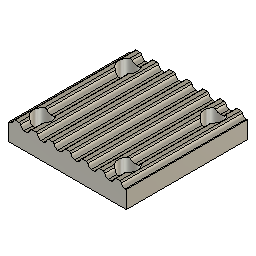
Carriage Rail Belt Clamp (Autodesk Fusion 360 archive; units mm, degrees)
design "TBCR Rail Belt Clamp" references "15mm HTD 5mm Timing Belt Loop"
Autodesk Fusion 360 part; units mm, degrees
(part 1 of 2)
sketch "Sketch1" plane through (0, 0, 0) normal (0, 0, 1) x (1, 0, 0)
  line L0 (17.5, 18) -> (-17.5, 18)
  line L1 (-17.5, 18) -> (-17.5, -18)
  line L2 (-17.5, -18) -> (17.5, -18)
  line L3 (17.5, -18) -> (17.5, 18)
  line L4 (17.5, 18) -> (-17.5, -18) construction
  line L5 (-17.5, 18) -> (17.5, -18) construction
  line L6 (0, 0) -> (0, 18) construction
  line L7 (0, 0) -> (17.5, 0) construction
  line L8 (12.5, 13) -> (-12.5, 13) construction
  line L9 (-12.5, 13) -> (-12.5, -13) construction
  line L10 (-12.5, -13) -> (12.5, -13) construction
  line L11 (12.5, -13) -> (12.5, 13) construction
  line L12 (12.5, 13) -> (-12.5, -13) construction
  line L13 (-12.5, 13) -> (12.5, -13) construction
  circle A0 centre (-12.5, 13) radius 2.25
  circle A1 centre (12.5, 13) radius 2.25
  circle A2 centre (12.5, -13) radius 2.25
  circle A3 centre (-12.5, -13) radius 2.25
  dimension "d10" = 35
  dimension "d11" = 36
  dimension "d13" = 25
  dimension "d14" = 26
  dimension "d15" = 4.5
  constraint horizontal L0
  constraint perpendicular L0 L1
  constraint parallel L0 L2
  constraint parallel L1 L3
  constraint coincident L4 L6.start
  constraint coincident L5 L6.start
  constraint coincident L6.start L7.start
  constraint midpoint L0 L6.end
  constraint midpoint L3 L7.end
  constraint horizontal L8
  constraint perpendicular L8 L9
  constraint parallel L8 L10
  constraint parallel L9 L11
  constraint coincident L12 L6.start
  constraint coincident L13 L6.start
  constraint coincident L8.end L9.start
  constraint coincident L8.start L11.end
  constraint coincident L10.end L11.start
  constraint coincident L9.end L10.start
  constraint equal A0 A3
  constraint equal A0 A2
  constraint equal A1 A2
  measures "d10" distance of L1.end L2.end
  measures "d11" distance of L0.end L1.end
  measures "d13" distance of L9.end L10.end
  measures "d14" distance of L8.end L9.end
  measures "d15" diameter of A0
extrude "Extrude1" add sketch "Sketch1" along normal blind 6.5
sketch "Sketch2" plane through (0, -18, 0) normal (0, -1, 0) x (1, 0, 0)
  line L0 (-17.5, 0) -> (17.5, 0)
  line L1 (17.5, 0) -> (17.5, 6.5)
  line L2 (17.5, 6.5) -> (-17.5, 6.5)
  line L3 (-17.5, 6.5) -> (-17.5, 0)
  arc A0 (-52.5, 8.4003) -> (-52.5, -87.0926) centre (-52.5, -39.3462) ccw
  line L4 (-52.5, -87.0926) -> (47.5, -87.0926)
  arc A1 (47.5, -87.0926) -> (47.5, 8.4003) centre (47.5, -39.3462) ccw
  line L5 (47.5, 8.4003) -> (-52.5, 8.4003)
  arc A2 (49.2562, -85.159) -> (50.5422, -85.0916) centre (47.5, -39.3462) ccw
  arc A3 (48.9524, -84.8176) -> (49.2562, -85.159) centre (49.4365, -84.6926) ccw
  arc A4 (48.9524, -84.8176) -> (47.9167, -83.7517) centre (47.5, -85.1926) ccw
  arc A5 (47.0833, -83.7517) -> (47.9167, -83.7517) centre (47.5, -83.03) ccw
  arc A6 (47.0833, -83.7517) -> (46.0476, -84.8176) centre (47.5, -85.1926) ccw
  arc A7 (45.5635, -85.1926) -> (46.0476, -84.8176) centre (45.5635, -84.6926) ccw
  line L6 (45.5635, -85.1926) -> (44.4365, -85.1926)
  arc A8 (43.9524, -84.8176) -> (44.4365, -85.1926) centre (44.4365, -84.6926) ccw
  arc A9 (43.9524, -84.8176) -> (42.9167, -83.7517) centre (42.5, -85.1926) ccw
  arc A10 (42.0833, -83.7517) -> (42.9167, -83.7517) centre (42.5, -83.03) ccw
  arc A11 (42.0833, -83.7517) -> (41.0476, -84.8176) centre (42.5, -85.1926) ccw
  arc A12 (40.5635, -85.1926) -> (41.0476, -84.8176) centre (40.5635, -84.6926) ccw
  line L7 (40.5635, -85.1926) -> (39.4365, -85.1926)
  arc A13 (38.9524, -84.8176) -> (39.4365, -85.1926) centre (39.4365, -84.6926) ccw
  arc A14 (38.9524, -84.8176) -> (37.9167, -83.7517) centre (37.5, -85.1926) ccw
  arc A15 (37.0833, -83.7517) -> (37.9167, -83.7517) centre (37.5, -83.03) ccw
  arc A16 (37.0833, -83.7517) -> (36.0476, -84.8176) centre (37.5, -85.1926) ccw
  arc A17 (35.5635, -85.1926) -> (36.0476, -84.8176) centre (35.5635, -84.6926) ccw
  line L8 (35.5635, -85.1926) -> (34.4365, -85.1926)
  arc A18 (33.9524, -84.8176) -> (34.4365, -85.1926) centre (34.4365, -84.6926) ccw
  arc A19 (33.9524, -84.8176) -> (32.9167, -83.7517) centre (32.5, -85.1926) ccw
  arc A20 (32.0833, -83.7517) -> (32.9167, -83.7517) centre (32.5, -83.03) ccw
  arc A21 (32.0833, -83.7517) -> (31.0476, -84.8176) centre (32.5, -85.1926) ccw
  arc A22 (30.5635, -85.1926) -> (31.0476, -84.8176) centre (30.5635, -84.6926) ccw
  line L9 (30.5635, -85.1926) -> (29.4365, -85.1926)
  arc A23 (28.9524, -84.8176) -> (29.4365, -85.1926) centre (29.4365, -84.6926) ccw
  arc A24 (28.9524, -84.8176) -> (27.9167, -83.7517) centre (27.5, -85.1926) ccw
  arc A25 (27.0833, -83.7517) -> (27.9167, -83.7517) centre (27.5, -83.03) ccw
  arc A26 (27.0833, -83.7517) -> (26.0476, -84.8176) centre (27.5, -85.1926) ccw
  arc A27 (25.5635, -85.1926) -> (26.0476, -84.8176) centre (25.5635, -84.6926) ccw
  line L10 (25.5635, -85.1926) -> (24.4365, -85.1926)
  arc A28 (23.9524, -84.8176) -> (24.4365, -85.1926) centre (24.4365, -84.6926) ccw
  arc A29 (23.9524, -84.8176) -> (22.9167, -83.7517) centre (22.5, -85.1926) ccw
  arc A30 (22.0833, -83.7517) -> (22.9167, -83.7517) centre (22.5, -83.03) ccw
  arc A31 (22.0833, -83.7517) -> (21.0476, -84.8176) centre (22.5, -85.1926) ccw
  arc A32 (20.5635, -85.1926) -> (21.0476, -84.8176) centre (20.5635, -84.6926) ccw
  line L11 (20.5635, -85.1926) -> (19.4365, -85.1926)
  arc A33 (18.9524, -84.8176) -> (19.4365, -85.1926) centre (19.4365, -84.6926) ccw
  arc A34 (18.9524, -84.8176) -> (17.9167, -83.7517) centre (17.5, -85.1926) ccw
  arc A35 (17.0833, -83.7517) -> (17.9167, -83.7517) centre (17.5, -83.03) ccw
  arc A36 (17.0833, -83.7517) -> (16.0476, -84.8176) centre (17.5, -85.1926) ccw
  arc A37 (15.5635, -85.1926) -> (16.0476, -84.8176) centre (15.5635, -84.6926) ccw
  line L12 (15.5635, -85.1926) -> (14.4365, -85.1926)
  arc A38 (13.9524, -84.8176) -> (14.4365, -85.1926) centre (14.4365, -84.6926) ccw
  arc A39 (13.9524, -84.8176) -> (12.9167, -83.7517) centre (12.5, -85.1926) ccw
  arc A40 (12.0833, -83.7517) -> (12.9167, -83.7517) centre (12.5, -83.03) ccw
  arc A41 (12.0833, -83.7517) -> (11.0476, -84.8176) centre (12.5, -85.1926) ccw
  arc A42 (10.5635, -85.1926) -> (11.0476, -84.8176) centre (10.5635, -84.6926) ccw
  line L13 (10.5635, -85.1926) -> (9.4365, -85.1926)
  arc A43 (8.9524, -84.8176) -> (9.4365, -85.1926) centre (9.4365, -84.6926) ccw
  arc A44 (8.9524, -84.8176) -> (7.9167, -83.7517) centre (7.5, -85.1926) ccw
  arc A45 (7.0833, -83.7517) -> (7.9167, -83.7517) centre (7.5, -83.03) ccw
  arc A46 (7.0833, -83.7517) -> (6.0476, -84.8176) centre (7.5, -85.1926) ccw
  arc A47 (5.5635, -85.1926) -> (6.0476, -84.8176) centre (5.5635, -84.6926) ccw
  line L14 (5.5635, -85.1926) -> (4.4365, -85.1926)
  arc A48 (3.9524, -84.8176) -> (4.4365, -85.1926) centre (4.4365, -84.6926) ccw
  arc A49 (3.9524, -84.8176) -> (2.9167, -83.7517) centre (2.5, -85.1926) ccw
  arc A50 (2.0833, -83.7517) -> (2.9167, -83.7517) centre (2.5, -83.03) ccw
  arc A51 (2.0833, -83.7517) -> (1.0476, -84.8176) centre (2.5, -85.1926) ccw
  arc A52 (0.5635, -85.1926) -> (1.0476, -84.8176) centre (0.5635, -84.6926) ccw
  line L15 (0.5635, -85.1926) -> (-0.5635, -85.1926)
  arc A53 (-1.0476, -84.8176) -> (-0.5635, -85.1926) centre (-0.5635, -84.6926) ccw
  arc A54 (-1.0476, -84.8176) -> (-2.0833, -83.7517) centre (-2.5, -85.1926) ccw
  arc A55 (-2.9167, -83.7517) -> (-2.0833, -83.7517) centre (-2.5, -83.03) ccw
  arc A56 (-2.9167, -83.7517) -> (-3.9524, -84.8176) centre (-2.5, -85.1926) ccw
  arc A57 (-4.4365, -85.1926) -> (-3.9524, -84.8176) centre (-4.4365, -84.6926) ccw
  line L16 (-4.4365, -85.1926) -> (-5.5635, -85.1926)
  arc A58 (-6.0476, -84.8176) -> (-5.5635, -85.1926) centre (-5.5635, -84.6926) ccw
  arc A59 (-6.0476, -84.8176) -> (-7.0833, -83.7517) centre (-7.5, -85.1926) ccw
  arc A60 (-7.9167, -83.7517) -> (-7.0833, -83.7517) centre (-7.5, -83.03) ccw
  arc A61 (-7.9167, -83.7517) -> (-8.9524, -84.8176) centre (-7.5, -85.1926) ccw
  arc A62 (-9.4365, -85.1926) -> (-8.9524, -84.8176) centre (-9.4365, -84.6926) ccw
  line L17 (-9.4365, -85.1926) -> (-10.5635, -85.1926)
  arc A63 (-11.0476, -84.8176) -> (-10.5635, -85.1926) centre (-10.5635, -84.6926) ccw
  arc A64 (-11.0476, -84.8176) -> (-12.0833, -83.7517) centre (-12.5, -85.1926) ccw
  arc A65 (-12.9167, -83.7517) -> (-12.0833, -83.7517) centre (-12.5, -83.03) ccw
  arc A66 (-12.9167, -83.7517) -> (-13.9524, -84.8176) centre (-12.5, -85.1926) ccw
  arc A67 (-14.4365, -85.1926) -> (-13.9524, -84.8176) centre (-14.4365, -84.6926) ccw
  line L18 (-14.4365, -85.1926) -> (-15.5635, -85.1926)
  arc A68 (-16.0476, -84.8176) -> (-15.5635, -85.1926) centre (-15.5635, -84.6926) ccw
  arc A69 (-16.0476, -84.8176) -> (-17.0833, -83.7517) centre (-17.5, -85.1926) ccw
  arc A70 (-17.9167, -83.7517) -> (-17.0833, -83.7517) centre (-17.5, -83.03) ccw
  arc A71 (-17.9167, -83.7517) -> (-18.9524, -84.8176) centre (-17.5, -85.1926) ccw
  arc A72 (-19.4365, -85.1926) -> (-18.9524, -84.8176) centre (-19.4365, -84.6926) ccw
  line L19 (-19.4365, -85.1926) -> (-20.5635, -85.1926)
  arc A73 (-21.0476, -84.8176) -> (-20.5635, -85.1926) centre (-20.5635, -84.6926) ccw
  arc A74 (-21.0476, -84.8176) -> (-22.0833, -83.7517) centre (-22.5, -85.1926) ccw
  arc A75 (-22.9167, -83.7517) -> (-22.0833, -83.7517) centre (-22.5, -83.03) ccw
  arc A76 (-22.9167, -83.7517) -> (-23.9524, -84.8176) centre (-22.5, -85.1926) ccw
  arc A77 (-24.4365, -85.1926) -> (-23.9524, -84.8176) centre (-24.4365, -84.6926) ccw
  line L20 (-24.4365, -85.1926) -> (-25.5635, -85.1926)
  arc A78 (-26.0476, -84.8176) -> (-25.5635, -85.1926) centre (-25.5635, -84.6926) ccw
  arc A79 (-26.0476, -84.8176) -> (-27.0833, -83.7517) centre (-27.5, -85.1926) ccw
  arc A80 (-27.9167, -83.7517) -> (-27.0833, -83.7517) centre (-27.5, -83.03) ccw
  arc A81 (-27.9167, -83.7517) -> (-28.9524, -84.8176) centre (-27.5, -85.1926) ccw
  arc A82 (-29.4365, -85.1926) -> (-28.9524, -84.8176) centre (-29.4365, -84.6926) ccw
  line L21 (-29.4365, -85.1926) -> (-30.5635, -85.1926)
  arc A83 (-31.0476, -84.8176) -> (-30.5635, -85.1926) centre (-30.5635, -84.6926) ccw
  arc A84 (-31.0476, -84.8176) -> (-32.0833, -83.7517) centre (-32.5, -85.1926) ccw
  arc A85 (-32.9167, -83.7517) -> (-32.0833, -83.7517) centre (-32.5, -83.03) ccw
  arc A86 (-32.9167, -83.7517) -> (-33.9524, -84.8176) centre (-32.5, -85.1926) ccw
  arc A87 (-34.4365, -85.1926) -> (-33.9524, -84.8176) centre (-34.4365, -84.6926) ccw
  line L22 (-34.4365, -85.1926) -> (-35.5635, -85.1926)
  arc A88 (-36.0476, -84.8176) -> (-35.5635, -85.1926) centre (-35.5635, -84.6926) ccw
  arc A89 (-36.0476, -84.8176) -> (-37.0833, -83.7517) centre (-37.5, -85.1926) ccw
  arc A90 (-37.9167, -83.7517) -> (-37.0833, -83.7517) centre (-37.5, -83.03) ccw
  arc A91 (-37.9167, -83.7517) -> (-38.9524, -84.8176) centre (-37.5, -85.1926) ccw
  arc A92 (-39.4365, -85.1926) -> (-38.9524, -84.8176) centre (-39.4365, -84.6926) ccw
  line L23 (-39.4365, -85.1926) -> (-40.5635, -85.1926)
  arc A93 (-41.0476, -84.8176) -> (-40.5635, -85.1926) centre (-40.5635, -84.6926) ccw
  arc A94 (-41.0476, -84.8176) -> (-42.0833, -83.7517) centre (-42.5, -85.1926) ccw
  arc A95 (-42.9167, -83.7517) -> (-42.0833, -83.7517) centre (-42.5, -83.03) ccw
  arc A96 (-42.9167, -83.7517) -> (-43.9524, -84.8176) centre (-42.5, -85.1926) ccw
  arc A97 (-44.4365, -85.1926) -> (-43.9524, -84.8176) centre (-44.4365, -84.6926) ccw
  line L24 (-44.4365, -85.1926) -> (-45.5635, -85.1926)
  arc A98 (-46.0476, -84.8176) -> (-45.5635, -85.1926) centre (-45.5635, -84.6926) ccw
  arc A99 (-46.0476, -84.8176) -> (-47.0833, -83.7517) centre (-47.5, -85.1926) ccw
  arc A100 (-47.9167, -83.7517) -> (-47.0833, -83.7517) centre (-47.5, -83.03) ccw
  arc A101 (-47.9167, -83.7517) -> (-48.9524, -84.8176) centre (-47.5, -85.1926) ccw
  arc A102 (-49.4365, -85.1926) -> (-48.9524, -84.8176) centre (-49.4365, -84.6926) ccw
  line L25 (-49.4365, -85.1926) -> (-50.5635, -85.1926)
  arc A103 (-51.0476, -84.8176) -> (-50.5635, -85.1926) centre (-50.5635, -84.6926) ccw
  arc A104 (-51.0476, -84.8176) -> (-52.0833, -83.7517) centre (-52.5, -85.1926) ccw
  arc A105 (-52.9167, -83.7517) -> (-52.0833, -83.7517) centre (-52.5, -83.03) ccw
  arc A106 (-52.9167, -83.7517) -> (-53.9524, -84.8176) centre (-52.5, -85.1926) ccw
  arc A107 (-54.2562, -85.159) -> (-53.9524, -84.8176) centre (-54.4365, -84.6926) ccw
  arc A108 (-55.5422, -85.0916) -> (-54.2562, -85.159) centre (-52.5, -39.3462) ccw
  arc A109 (-55.8087, -84.7204) -> (-55.5422, -85.0916) centre (-55.3141, -84.6466) ccw
  arc A110 (-55.8087, -84.7204) -> (-56.7273, -83.552) centre (-57.2923, -84.9415) ccw
  arc A111 (-57.556, -83.4649) -> (-56.7273, -83.552) centre (-57.0662, -82.7907) ccw
  arc A112 (-57.556, -83.4649) -> (-58.6975, -84.4167) centre (-57.2923, -84.9415) ccw
  arc A113 (-59.0353, -84.7245) -> (-58.6975, -84.4167) centre (-59.1659, -84.2418) ccw
  arc A114 (-60.3072, -84.523) -> (-59.0353, -84.7245) centre (-52.5, -39.3462) ccw
  arc A115 (-60.5334, -84.1259) -> (-60.3072, -84.523) centre (-60.0339, -84.1043) ccw
  arc A116 (-60.5334, -84.1259) -> (-61.3249, -82.8679) centre (-62.032, -84.1908) ccw
  arc A117 (-62.14, -82.6947) -> (-61.3249, -82.8679) centre (-61.5824, -82.0754) ccw
  arc A118 (-62.14, -82.6947) -> (-63.3747, -83.522) centre (-62.032, -84.1908) ccw
  arc A119 (-63.7428, -83.7927) -> (-63.3747, -83.522) centre (-63.8222, -83.2991) ccw
  arc A120 (-64.9867, -83.4594) -> (-63.7428, -83.7927) centre (-52.5, -39.3462) ccw
  arc A121 (-65.1702, -83.0409) -> (-64.9867, -83.4594) centre (-64.6711, -83.0716) ccw
  arc A122 (-65.1702, -83.0409) -> (-65.8258, -81.7071) centre (-66.6673, -82.9488) ccw
  arc A123 (-66.6183, -81.4496) -> (-65.8258, -81.7071) centre (-65.999, -80.8919) ccw
  arc A124 (-66.6183, -81.4496) -> (-67.9327, -82.1433) centre (-66.6673, -82.9488) ccw
  arc A125 (-68.3272, -82.3741) -> (-67.9327, -82.1433) centre (-68.3545, -81.8748) ccw
  arc A126 (-69.5294, -81.9126) -> (-68.3272, -82.3741) centre (-52.5, -39.3462) ccw
  arc A127 (-69.6681, -81.4772) -> (-69.5294, -81.9126) centre (-69.175, -81.5599) ccw
  arc A128 (-69.6681, -81.4772) -> (-70.1807, -80.0821) centre (-71.1474, -81.229) ccw
  arc A129 (-70.942, -79.7431) -> (-70.1807, -80.0821) centre (-70.2678, -79.2533) ccw
  arc A130 (-70.942, -79.7431) -> (-72.3217, -80.2957) centre (-71.1474, -81.229) ccw
  arc A131 (-72.7381, -80.484) -> (-72.3217, -80.2957) centre (-72.7131, -79.9846) ccw
  arc A132 (-73.8855, -79.8993) -> (-72.7381, -80.484) centre (-52.5, -39.3462) ccw
  arc A133 (-73.978, -79.4518) -> (-73.8855, -79.8993) centre (-73.4962, -79.5856) ccw
  arc A134 (-73.978, -79.4518) -> (-74.3419, -78.0108) centre (-75.4232, -79.0504) ccw
  arc A135 (-75.0636, -77.5941) -> (-74.3419, -78.0108) centre (-74.3419, -77.1775) ccw
  arc A136 (-75.0636, -77.5941) -> (-76.4935, -77.9994) centre (-75.4232, -79.0504) ccw
  arc A137 (-76.9273, -78.1432) -> (-76.4935, -77.9994) centre (-76.8503, -77.6491) ccw
  arc A138 (-78.0073, -77.4418) -> (-76.9273, -78.1432) centre (-52.5, -39.3462) ccw
  arc A139 (-78.0525, -76.987) -> (-78.0073, -77.4418) centre (-77.5873, -77.1705) ccw
  arc A140 (-78.0525, -76.987) -> (-78.2638, -75.5159) centre (-79.4479, -76.4367) ccw
  arc A141 (-78.938, -75.0261) -> (-78.2638, -75.5159) centre (-78.1767, -74.6871) ccw
  arc A142 (-78.938, -75.0261) -> (-80.4025, -75.2797) centre (-79.4479, -76.4367) ccw
  arc A143 (-80.8489, -75.3773) -> (-80.4025, -75.2797) centre (-80.7206, -74.894) ccw
  arc A144 (-81.8497, -74.5668) -> (-80.8489, -75.3773) centre (-52.5, -39.3462) ccw
  arc A145 (-81.847, -74.1099) -> (-81.8497, -74.5668) centre (-81.4036, -74.3409) ccw
  arc A146 (-81.847, -74.1099) -> (-81.9034, -72.6247) centre (-83.1773, -73.4167) ccw
  arc A147 (-82.5227, -72.0671) -> (-81.9034, -72.6247) centre (-81.7302, -71.8096) ccw
  arc A148 (-82.5227, -72.0671) -> (-84.0057, -72.1662) centre (-83.1773, -73.4167) ccw
  arc A149 (-84.4599, -72.2166) -> (-84.0057, -72.1662) centre (-84.2818, -71.7494) ccw
  arc A150 (-85.3705, -71.306) -> (-84.4599, -72.2166) centre (-52.5, -39.3462) ccw
  arc A151 (-85.3201, -70.8518) -> (-85.3705, -71.306) centre (-84.9032, -71.128) ccw
  arc A152 (-85.3201, -70.8518) -> (-85.2209, -69.3689) centre (-86.5706, -70.0234) ccw
  arc A153 (-85.7785, -68.7496) -> (-85.2209, -69.3689) centre (-84.9634, -68.5763) ccw
  arc A154 (-85.7785, -68.7496) -> (-87.2637, -68.6932) centre (-86.5706, -70.0234) ccw
  arc A155 (-87.7207, -68.6958) -> (-87.2637, -68.6932) centre (-87.4948, -68.2498) ccw
  arc A156 (-88.5311, -67.695) -> (-87.7207, -68.6958) centre (-52.5, -39.3462) ccw
  arc A157 (-88.4335, -67.2486) -> (-88.5311, -67.695) centre (-88.0478, -67.5668) ccw
  arc A158 (-88.4335, -67.2486) -> (-88.1799, -65.7842) centre (-89.5906, -66.294) ccw
  arc A159 (-88.6697, -65.11) -> (-88.1799, -65.7842) centre (-87.841, -65.0229) ccw
  arc A160 (-88.6697, -65.11) -> (-90.1409, -64.8986) centre (-89.5906, -66.294) ccw
  arc A161 (-90.5956, -64.8535) -> (-90.1409, -64.8986) centre (-90.3243, -64.4335) ccw
  arc A162 (-91.297, -63.7735) -> (-90.5956, -64.8535) centre (-52.5, -39.3462) ccw
  arc A163 (-91.1533, -63.3397) -> (-91.297, -63.7735) centre (-90.803, -63.6965) ccw
  arc A164 (-91.1533, -63.3397) -> (-90.748, -61.9098) centre (-92.2042, -62.2694) ccw
  arc A165 (-91.1646, -61.1881) -> (-90.748, -61.9098) centre (-90.3313, -61.1881) ccw
  arc A166 (-91.1646, -61.1881) -> (-92.6056, -60.8241) centre (-92.2042, -62.2694) ccw
  arc A167 (-93.0532, -60.7317) -> (-92.6056, -60.8241) centre (-92.7395, -60.3424) ccw
  arc A168 (-93.6378, -59.5843) -> (-93.0532, -60.7317) centre (-52.5, -39.3462) ccw
  arc A169 (-93.4495, -59.1679) -> (-93.6378, -59.5843) centre (-93.1384, -59.5593) ccw
  arc A170 (-93.4495, -59.1679) -> (-92.897, -57.7882) centre (-94.3828, -57.9936) ccw
  arc A171 (-93.2359, -57.0269) -> (-92.897, -57.7882) centre (-92.4072, -57.114) ccw
  arc A172 (-93.2359, -57.0269) -> (-94.631, -56.5143) centre (-94.3828, -57.9936) ccw
  arc A173 (-95.0664, -56.3756) -> (-94.631, -56.5143) centre (-94.7137, -56.0212) ccw
  arc A174 (-95.5279, -55.1733) -> (-95.0664, -56.3756) centre (-52.5, -39.3462) ccw
  arc A175 (-95.2971, -54.7789) -> (-95.5279, -55.1733) centre (-95.0287, -55.2007) ccw
  arc A176 (-95.2971, -54.7789) -> (-94.6034, -53.4645) centre (-96.1026, -53.5135) ccw
  arc A177 (-94.8609, -52.6719) -> (-94.6034, -53.4645) centre (-94.0458, -52.8452) ccw
  arc A178 (-94.8609, -52.6719) -> (-96.1948, -52.0163) centre (-96.1026, -53.5135) ccw
  arc A179 (-96.6133, -51.8329) -> (-96.1948, -52.0163) centre (-96.2255, -51.5173) ccw
  arc A180 (-96.9466, -50.589) -> (-96.6133, -51.8329) centre (-52.5, -39.3462) ccw
  arc A181 (-96.6759, -50.2208) -> (-96.9466, -50.589) centre (-96.4529, -50.6684) ccw
  arc A182 (-96.6759, -50.2208) -> (-95.8485, -48.9861) centre (-97.3446, -48.8782) ccw
  arc A183 (-96.0218, -48.171) -> (-95.8485, -48.9861) centre (-95.2292, -48.4285) ccw
  arc A184 (-96.0218, -48.171) -> (-97.2798, -47.3796) centre (-97.3446, -48.8782) ccw
  arc A185 (-97.6768, -47.1534) -> (-97.2798, -47.3796) centre (-97.2582, -46.88) ccw
  arc A186 (-97.8783, -45.8815) -> (-97.6768, -47.1534) centre (-52.5, -39.3462) ccw
  arc A187 (-97.5706, -45.5436) -> (-97.8783, -45.8815) centre (-97.3957, -46.012) ccw
  arc A188 (-97.5706, -45.5436) -> (-96.6187, -44.4022) centre (-98.0953, -44.1384) ccw
  arc A189 (-96.7058, -43.5734) -> (-96.6187, -44.4022) centre (-95.9445, -43.9124) ccw
  arc A190 (-96.7058, -43.5734) -> (-97.8742, -42.6548) centre (-98.0953, -44.1384) ccw
  arc A191 (-98.2454, -42.3884) -> (-97.8742, -42.6548) centre (-97.8005, -42.1603) ccw
  arc A192 (-98.3128, -41.1023) -> (-98.2454, -42.3884) centre (-52.5, -39.3462) ccw
  arc A193 (-97.9715, -40.7985) -> (-98.3128, -41.1023) centre (-97.8465, -41.2827) ccw
  arc A194 (-97.9715, -40.7985) -> (-96.9055, -39.7628) centre (-98.3465, -39.3462) ccw
  arc A195 (-96.9055, -38.9295) -> (-96.9055, -39.7628) centre (-96.1838, -39.3462) ccw
  arc A196 (-96.9055, -38.9295) -> (-97.9715, -37.8938) centre (-98.3465, -39.3462) ccw
  arc A197 (-98.3128, -37.59) -> (-97.9715, -37.8938) centre (-97.8465, -37.4097) ccw
  arc A198 (-98.2454, -36.304) -> (-98.3128, -37.59) centre (-52.5, -39.3462) ccw
  arc A199 (-97.8742, -36.0375) -> (-98.2454, -36.304) centre (-97.8005, -36.532) ccw
  arc A200 (-97.8742, -36.0375) -> (-96.7058, -35.1189) centre (-98.0953, -34.5539) ccw
  arc A201 (-96.6187, -34.2901) -> (-96.7058, -35.1189) centre (-95.9445, -34.78) ccw
  arc A202 (-96.6187, -34.2901) -> (-97.5706, -33.1487) centre (-98.0953, -34.5539) ccw
  arc A203 (-97.8783, -32.8109) -> (-97.5706, -33.1487) centre (-97.3957, -32.6803) ccw
  arc A204 (-97.6768, -31.5389) -> (-97.8783, -32.8109) centre (-52.5, -39.3462) ccw
  arc A205 (-97.2798, -31.3127) -> (-97.6768, -31.5389) centre (-97.2582, -31.8123) ccw
  arc A206 (-97.2798, -31.3127) -> (-96.0218, -30.5213) centre (-97.3446, -29.8141) ccw
  arc A207 (-95.8485, -29.7062) -> (-96.0218, -30.5213) centre (-95.2292, -30.2638) ccw
  arc A208 (-95.8485, -29.7062) -> (-96.6759, -28.4715) centre (-97.3446, -29.8141) ccw
  arc A209 (-96.9466, -28.1033) -> (-96.6759, -28.4715) centre (-96.4529, -28.0239) ccw
  arc A210 (-96.6133, -26.8594) -> (-96.9466, -28.1033) centre (-52.5, -39.3462) ccw
  arc A211 (-96.1948, -26.676) -> (-96.6133, -26.8594) centre (-96.2255, -27.175) ccw
  arc A212 (-96.1948, -26.676) -> (-94.8609, -26.0204) centre (-96.1026, -25.1788) ccw
  arc A213 (-94.6034, -25.2278) -> (-94.8609, -26.0204) centre (-94.0458, -25.8471) ccw
  arc A214 (-94.6034, -25.2278) -> (-95.2971, -23.9134) centre (-96.1026, -25.1788) ccw
  arc A215 (-95.5279, -23.519) -> (-95.2971, -23.9134) centre (-95.0287, -23.4916) ccw
  arc A216 (-95.0664, -22.3167) -> (-95.5279, -23.519) centre (-52.5, -39.3462) ccw
  arc A217 (-94.631, -22.178) -> (-95.0664, -22.3167) centre (-94.7137, -22.6712) ccw
  arc A218 (-94.631, -22.178) -> (-93.2359, -21.6655) centre (-94.3828, -20.6987) ccw
  arc A219 (-92.897, -20.9042) -> (-93.2359, -21.6655) centre (-92.4072, -21.5783) ccw
  arc A220 (-92.897, -20.9042) -> (-93.4495, -19.5244) centre (-94.3828, -20.6987) ccw
  arc A221 (-93.6378, -19.1081) -> (-93.4495, -19.5244) centre (-93.1384, -19.133) ccw
  arc A222 (-93.0532, -17.9606) -> (-93.6378, -19.1081) centre (-52.5, -39.3462) ccw
  arc A223 (-92.6056, -17.8682) -> (-93.0532, -17.9606) centre (-92.7395, -18.35) ccw
  arc A224 (-92.6056, -17.8682) -> (-91.1646, -17.5042) centre (-92.2042, -16.4229) ccw
  arc A225 (-90.748, -16.7826) -> (-91.1646, -17.5042) centre (-90.3313, -17.5042) ccw
  arc A226 (-90.748, -16.7826) -> (-91.1533, -15.3526) centre (-92.2042, -16.4229) ccw
  arc A227 (-91.297, -14.9189) -> (-91.1533, -15.3526) centre (-90.803, -14.9959) ccw
  arc A228 (-90.5956, -13.8388) -> (-91.297, -14.9189) centre (-52.5, -39.3462) ccw
  arc A229 (-90.1409, -13.7937) -> (-90.5956, -13.8388) centre (-90.3243, -14.2588) ccw
  arc A230 (-90.1409, -13.7937) -> (-88.6697, -13.5823) centre (-89.5906, -12.3983) ccw
  arc A231 (-88.1799, -12.9082) -> (-88.6697, -13.5823) centre (-87.841, -13.6695) ccw
  arc A232 (-88.1799, -12.9082) -> (-88.4335, -11.4437) centre (-89.5906, -12.3983) ccw
  arc A233 (-88.5311, -10.9973) -> (-88.4335, -11.4437) centre (-88.0478, -11.1255) ccw
  arc A234 (-87.7207, -9.9965) -> (-88.5311, -10.9973) centre (-52.5, -39.3462) ccw
  arc A235 (-87.2637, -9.9991) -> (-87.7207, -9.9965) centre (-87.4948, -10.4425) ccw
  arc A236 (-87.2637, -9.9991) -> (-85.7785, -9.9427) centre (-86.5706, -8.6689) ccw
  arc A237 (-85.2209, -9.3234) -> (-85.7785, -9.9427) centre (-84.9634, -10.116) ccw
  arc A238 (-85.2209, -9.3234) -> (-85.3201, -7.8405) centre (-86.5706, -8.6689) ccw
  arc A239 (-85.3705, -7.3863) -> (-85.3201, -7.8405) centre (-84.9032, -7.5643) ccw
  arc A240 (-84.4599, -6.4757) -> (-85.3705, -7.3863) centre (-52.5, -39.3462) ccw
  arc A241 (-84.0057, -6.5261) -> (-84.4599, -6.4757) centre (-84.2818, -6.9429) ccw
  arc A242 (-84.0057, -6.5261) -> (-82.5227, -6.6252) centre (-83.1773, -5.2756) ccw
  arc A243 (-81.9034, -6.0676) -> (-82.5227, -6.6252) centre (-81.7302, -6.8828) ccw
  arc A244 (-81.9034, -6.0676) -> (-81.847, -4.5824) centre (-83.1773, -5.2756) ccw
  arc A245 (-81.8497, -4.1255) -> (-81.847, -4.5824) centre (-81.4036, -4.3514) ccw
  arc A246 (-80.8489, -3.315) -> (-81.8497, -4.1255) centre (-52.5, -39.3462) ccw
  arc A247 (-80.4025, -3.4126) -> (-80.8489, -3.315) centre (-80.7206, -3.7983) ccw
  arc A248 (-80.4025, -3.4126) -> (-78.938, -3.6663) centre (-79.4479, -2.2556) ccw
  arc A249 (-78.2638, -3.1764) -> (-78.938, -3.6663) centre (-78.1767, -4.0052) ccw
  arc A250 (-78.2638, -3.1764) -> (-78.0525, -1.7053) centre (-79.4479, -2.2556) ccw
  arc A251 (-78.0073, -1.2505) -> (-78.0525, -1.7053) centre (-77.5873, -1.5218) ccw
  arc A252 (-76.9273, -0.5492) -> (-78.0073, -1.2505) centre (-52.5, -39.3462) ccw
  arc A253 (-76.4935, -0.6929) -> (-76.9273, -0.5492) centre (-76.8503, -1.0432) ccw
  arc A254 (-76.4935, -0.6929) -> (-75.0636, -1.0982) centre (-75.4232, 0.3581) ccw
  arc A255 (-74.3419, -0.6815) -> (-75.0636, -1.0982) centre (-74.3419, -1.5149) ccw
  arc A256 (-74.3419, -0.6815) -> (-73.978, 0.7595) centre (-75.4232, 0.3581) ccw
  arc A257 (-73.8855, 1.207) -> (-73.978, 0.7595) centre (-73.4962, 0.8933) ccw
  arc A258 (-72.7381, 1.7916) -> (-73.8855, 1.207) centre (-52.5, -39.3462) ccw
  arc A259 (-72.3217, 1.6034) -> (-72.7381, 1.7916) centre (-72.7131, 1.2923) ccw
  arc A260 (-72.3217, 1.6034) -> (-70.942, 1.0508) centre (-71.1474, 2.5367) ccw
  arc A261 (-70.1807, 1.3898) -> (-70.942, 1.0508) centre (-70.2678, 0.561) ccw
  arc A262 (-70.1807, 1.3898) -> (-69.6681, 2.7848) centre (-71.1474, 2.5367) ccw
  arc A263 (-69.5294, 3.2202) -> (-69.6681, 2.7848) centre (-69.175, 2.8676) ccw
  arc A264 (-68.3272, 3.6817) -> (-69.5294, 3.2202) centre (-52.5, -39.3462) ccw
  arc A265 (-67.9327, 3.451) -> (-68.3272, 3.6817) centre (-68.3545, 3.1825) ccw
  arc A266 (-67.9327, 3.451) -> (-66.6183, 2.7572) centre (-66.6673, 4.2564) ccw
  arc A267 (-65.8258, 3.0148) -> (-66.6183, 2.7572) centre (-65.999, 2.1996) ccw
  arc A268 (-65.8258, 3.0148) -> (-65.1702, 4.3486) centre (-66.6673, 4.2564) ccw
  arc A269 (-64.9867, 4.7671) -> (-65.1702, 4.3486) centre (-64.6711, 4.3793) ccw
  arc A270 (-63.7428, 5.1004) -> (-64.9867, 4.7671) centre (-52.5, -39.3462) ccw
  arc A271 (-63.3747, 4.8297) -> (-63.7428, 5.1004) centre (-63.8222, 4.6068) ccw
  arc A272 (-63.3747, 4.8297) -> (-62.14, 4.0024) centre (-62.032, 5.4985) ccw
  arc A273 (-61.3249, 4.1756) -> (-62.14, 4.0024) centre (-61.5824, 3.3831) ccw
  arc A274 (-61.3249, 4.1756) -> (-60.5334, 5.4336) centre (-62.032, 5.4985) ccw
  arc A275 (-60.3072, 5.8307) -> (-60.5334, 5.4336) centre (-60.0339, 5.412) ccw
  arc A276 (-59.0353, 6.0321) -> (-60.3072, 5.8307) centre (-52.5, -39.3462) ccw
  arc A277 (-58.6975, 5.7244) -> (-59.0353, 6.0321) centre (-59.1659, 5.5495) ccw
  arc A278 (-58.6975, 5.7244) -> (-57.556, 4.7725) centre (-57.2923, 6.2492) ccw
  arc A279 (-56.7273, 4.8596) -> (-57.556, 4.7725) centre (-57.0662, 4.0984) ccw
  arc A280 (-56.7273, 4.8596) -> (-55.8087, 6.028) centre (-57.2923, 6.2492) ccw
  arc A281 (-55.5422, 6.3993) -> (-55.8087, 6.028) centre (-55.3141, 5.9543) ccw
  arc A282 (-54.2562, 6.4667) -> (-55.5422, 6.3993) centre (-52.5, -39.3462) ccw
  arc A283 (-53.9524, 6.1253) -> (-54.2562, 6.4667) centre (-54.4365, 6.0003) ccw
  arc A284 (-53.9524, 6.1253) -> (-52.9167, 5.0594) centre (-52.5, 6.5003) ccw
  arc A285 (-52.0833, 5.0594) -> (-52.9167, 5.0594) centre (-52.5, 4.3377) ccw
  arc A286 (-52.0833, 5.0594) -> (-51.0476, 6.1253) centre (-52.5, 6.5003) ccw
  arc A287 (-50.5635, 6.5003) -> (-51.0476, 6.1253) centre (-50.5635, 6.0003) ccw
  line L26 (-50.5635, 6.5003) -> (-49.4365, 6.5003)
  arc A288 (-48.9524, 6.1253) -> (-49.4365, 6.5003) centre (-49.4365, 6.0003) ccw
  arc A289 (-48.9524, 6.1253) -> (-47.9167, 5.0594) centre (-47.5, 6.5003) ccw
  arc A290 (-47.0833, 5.0594) -> (-47.9167, 5.0594) centre (-47.5, 4.3377) ccw
  arc A291 (-47.0833, 5.0594) -> (-46.0476, 6.1253) centre (-47.5, 6.5003) ccw
  arc A292 (-45.5635, 6.5003) -> (-46.0476, 6.1253) centre (-45.5635, 6.0003) ccw
  line L27 (-45.5635, 6.5003) -> (-44.4365, 6.5003)
  arc A293 (-43.9524, 6.1253) -> (-44.4365, 6.5003) centre (-44.4365, 6.0003) ccw
  arc A294 (-43.9524, 6.1253) -> (-42.9167, 5.0594) centre (-42.5, 6.5003) ccw
  arc A295 (-42.0833, 5.0594) -> (-42.9167, 5.0594) centre (-42.5, 4.3377) ccw
  arc A296 (-42.0833, 5.0594) -> (-41.0476, 6.1253) centre (-42.5, 6.5003) ccw
  arc A297 (-40.5635, 6.5003) -> (-41.0476, 6.1253) centre (-40.5635, 6.0003) ccw
  line L28 (-40.5635, 6.5003) -> (-39.4365, 6.5003)
  arc A298 (-38.9524, 6.1253) -> (-39.4365, 6.5003) centre (-39.4365, 6.0003) ccw
  arc A299 (-38.9524, 6.1253) -> (-37.9167, 5.0594) centre (-37.5, 6.5003) ccw
  arc A300 (-37.0833, 5.0594) -> (-37.9167, 5.0594) centre (-37.5, 4.3377) ccw
  arc A301 (-37.0833, 5.0594) -> (-36.0476, 6.1253) centre (-37.5, 6.5003) ccw
  arc A302 (-35.5635, 6.5003) -> (-36.0476, 6.1253) centre (-35.5635, 6.0003) ccw
  line L29 (-35.5635, 6.5003) -> (-34.4365, 6.5003)
  arc A303 (-33.9524, 6.1253) -> (-34.4365, 6.5003) centre (-34.4365, 6.0003) ccw
  arc A304 (-33.9524, 6.1253) -> (-32.9167, 5.0594) centre (-32.5, 6.5003) ccw
  arc A305 (-32.0833, 5.0594) -> (-32.9167, 5.0594) centre (-32.5, 4.3377) ccw
  arc A306 (-32.0833, 5.0594) -> (-31.0476, 6.1253) centre (-32.5, 6.5003) ccw
  arc A307 (-30.5635, 6.5003) -> (-31.0476, 6.1253) centre (-30.5635, 6.0003) ccw
  line L30 (-30.5635, 6.5003) -> (-29.4365, 6.5003)
  arc A308 (-28.9524, 6.1253) -> (-29.4365, 6.5003) centre (-29.4365, 6.0003) ccw
  arc A309 (-28.9524, 6.1253) -> (-27.9167, 5.0594) centre (-27.5, 6.5003) ccw
  arc A310 (-27.0833, 5.0594) -> (-27.9167, 5.0594) centre (-27.5, 4.3377) ccw
  arc A311 (-27.0833, 5.0594) -> (-26.0476, 6.1253) centre (-27.5, 6.5003) ccw
  arc A312 (-25.5635, 6.5003) -> (-26.0476, 6.1253) centre (-25.5635, 6.0003) ccw
  line L31 (-25.5635, 6.5003) -> (-24.4365, 6.5003)
  arc A313 (-23.9524, 6.1253) -> (-24.4365, 6.5003) centre (-24.4365, 6.0003) ccw
  arc A314 (-23.9524, 6.1253) -> (-22.9167, 5.0594) centre (-22.5, 6.5003) ccw
  arc A315 (-22.0833, 5.0594) -> (-22.9167, 5.0594) centre (-22.5, 4.3377) ccw
  arc A316 (-22.0833, 5.0594) -> (-21.0476, 6.1253) centre (-22.5, 6.5003) ccw
  arc A317 (-20.5635, 6.5003) -> (-21.0476, 6.1253) centre (-20.5635, 6.0003) ccw
  line L32 (-20.5635, 6.5003) -> (-19.4365, 6.5003)
  arc A318 (-18.9524, 6.1253) -> (-19.4365, 6.5003) centre (-19.4365, 6.0003) ccw
  arc A319 (-18.9524, 6.1253) -> (-17.9167, 5.0594) centre (-17.5, 6.5003) ccw
  arc A320 (-17.0833, 5.0594) -> (-17.9167, 5.0594) centre (-17.5, 4.3377) ccw
  arc A321 (-17.0833, 5.0594) -> (-16.0476, 6.1253) centre (-17.5, 6.5003) ccw
  arc A322 (-15.5635, 6.5003) -> (-16.0476, 6.1253) centre (-15.5635, 6.0003) ccw
  line L33 (-15.5635, 6.5003) -> (-14.4365, 6.5003)
  arc A323 (-13.9524, 6.1253) -> (-14.4365, 6.5003) centre (-14.4365, 6.0003) ccw
  arc A324 (-13.9524, 6.1253) -> (-12.9167, 5.0594) centre (-12.5, 6.5003) ccw
  arc A325 (-12.0833, 5.0594) -> (-12.9167, 5.0594) centre (-12.5, 4.3377) ccw
  arc A326 (-12.0833, 5.0594) -> (-11.0476, 6.1253) centre (-12.5, 6.5003) ccw
  arc A327 (-10.5635, 6.5003) -> (-11.0476, 6.1253) centre (-10.5635, 6.0003) ccw
  line L34 (-10.5635, 6.5003) -> (-9.4365, 6.5003)
  arc A328 (-8.9524, 6.1253) -> (-9.4365, 6.5003) centre (-9.4365, 6.0003) ccw
  arc A329 (-8.9524, 6.1253) -> (-7.9167, 5.0594) centre (-7.5, 6.5003) ccw
  arc A330 (-7.0833, 5.0594) -> (-7.9167, 5.0594) centre (-7.5, 4.3377) ccw
  arc A331 (-7.0833, 5.0594) -> (-6.0476, 6.1253) centre (-7.5, 6.5003) ccw
  arc A332 (-5.5635, 6.5003) -> (-6.0476, 6.1253) centre (-5.5635, 6.0003) ccw
  line L35 (-5.5635, 6.5003) -> (-4.4365, 6.5003)
  arc A333 (-3.9524, 6.1253) -> (-4.4365, 6.5003) centre (-4.4365, 6.0003) ccw
  arc A334 (-3.9524, 6.1253) -> (-2.9167, 5.0594) centre (-2.5, 6.5003) ccw
  arc A335 (-2.0833, 5.0594) -> (-2.9167, 5.0594) centre (-2.5, 4.3377) ccw
  arc A336 (-2.0833, 5.0594) -> (-1.0476, 6.1253) centre (-2.5, 6.5003) ccw
  arc A337 (-0.5635, 6.5003) -> (-1.0476, 6.1253) centre (-0.5635, 6.0003) ccw
  line L36 (-0.5635, 6.5003) -> (0.5635, 6.5003)
  arc A338 (1.0476, 6.1253) -> (0.5635, 6.5003) centre (0.5635, 6.0003) ccw
  arc A339 (1.0476, 6.1253) -> (2.0833, 5.0594) centre (2.5, 6.5003) ccw
  arc A340 (2.9167, 5.0594) -> (2.0833, 5.0594) centre (2.5, 4.3377) ccw
  arc A341 (2.9167, 5.0594) -> (3.9524, 6.1253) centre (2.5, 6.5003) ccw
  arc A342 (4.4365, 6.5003) -> (3.9524, 6.1253) centre (4.4365, 6.0003) ccw
  line L37 (4.4365, 6.5003) -> (5.5635, 6.5003)
  arc A343 (6.0476, 6.1253) -> (5.5635, 6.5003) centre (5.5635, 6.0003) ccw
  arc A344 (6.0476, 6.1253) -> (7.0833, 5.0594) centre (7.5, 6.5003) ccw
  arc A345 (7.9167, 5.0594) -> (7.0833, 5.0594) centre (7.5, 4.3377) ccw
  arc A346 (7.9167, 5.0594) -> (8.9524, 6.1253) centre (7.5, 6.5003) ccw
  arc A347 (9.4365, 6.5003) -> (8.9524, 6.1253) centre (9.4365, 6.0003) ccw
  line L38 (9.4365, 6.5003) -> (10.5635, 6.5003)
  arc A348 (11.0476, 6.1253) -> (10.5635, 6.5003) centre (10.5635, 6.0003) ccw
  arc A349 (11.0476, 6.1253) -> (12.0833, 5.0594) centre (12.5, 6.5003) ccw
  arc A350 (12.9167, 5.0594) -> (12.0833, 5.0594) centre (12.5, 4.3377) ccw
  arc A351 (12.9167, 5.0594) -> (13.9524, 6.1253) centre (12.5, 6.5003) ccw
  arc A352 (14.4365, 6.5003) -> (13.9524, 6.1253) centre (14.4365, 6.0003) ccw
  line L39 (14.4365, 6.5003) -> (15.5635, 6.5003)
  arc A353 (16.0476, 6.1253) -> (15.5635, 6.5003) centre (15.5635, 6.0003) ccw
  arc A354 (16.0476, 6.1253) -> (17.0833, 5.0594) centre (17.5, 6.5003) ccw
  arc A355 (17.9167, 5.0594) -> (17.0833, 5.0594) centre (17.5, 4.3377) ccw
  arc A356 (17.9167, 5.0594) -> (18.9524, 6.1253) centre (17.5, 6.5003) ccw
  arc A357 (19.4365, 6.5003) -> (18.9524, 6.1253) centre (19.4365, 6.0003) ccw
  line L40 (19.4365, 6.5003) -> (20.5635, 6.5003)
  arc A358 (21.0476, 6.1253) -> (20.5635, 6.5003) centre (20.5635, 6.0003) ccw
  arc A359 (21.0476, 6.1253) -> (22.0833, 5.0594) centre (22.5, 6.5003) ccw
  arc A360 (22.9167, 5.0594) -> (22.0833, 5.0594) centre (22.5, 4.3377) ccw
  arc A361 (22.9167, 5.0594) -> (23.9524, 6.1253) centre (22.5, 6.5003) ccw
  arc A362 (24.4365, 6.5003) -> (23.9524, 6.1253) centre (24.4365, 6.0003) ccw
  line L41 (24.4365, 6.5003) -> (25.5635, 6.5003)
  arc A363 (26.0476, 6.1253) -> (25.5635, 6.5003) centre (25.5635, 6.0003) ccw
  arc A364 (26.0476, 6.1253) -> (27.0833, 5.0594) centre (27.5, 6.5003) ccw
  arc A365 (27.9167, 5.0594) -> (27.0833, 5.0594) centre (27.5, 4.3377) ccw
  arc A366 (27.9167, 5.0594) -> (28.9524, 6.1253) centre (27.5, 6.5003) ccw
  arc A367 (29.4365, 6.5003) -> (28.9524, 6.1253) centre (29.4365, 6.0003) ccw
  line L42 (29.4365, 6.5003) -> (30.5635, 6.5003)
  arc A368 (31.0476, 6.1253) -> (30.5635, 6.5003) centre (30.5635, 6.0003) ccw
  arc A369 (31.0476, 6.1253) -> (32.0833, 5.0594) centre (32.5, 6.5003) ccw
  arc A370 (32.9167, 5.0594) -> (32.0833, 5.0594) centre (32.5, 4.3377) ccw
  arc A371 (32.9167, 5.0594) -> (33.9524, 6.1253) centre (32.5, 6.5003) ccw
  arc A372 (34.4365, 6.5003) -> (33.9524, 6.1253) centre (34.4365, 6.0003) ccw
  line L43 (34.4365, 6.5003) -> (35.5635, 6.5003)
  arc A373 (36.0476, 6.1253) -> (35.5635, 6.5003) centre (35.5635, 6.0003) ccw
  arc A374 (36.0476, 6.1253) -> (37.0833, 5.0594) centre (37.5, 6.5003) ccw
  arc A375 (37.9167, 5.0594) -> (37.0833, 5.0594) centre (37.5, 4.3377) ccw
  arc A376 (37.9167, 5.0594) -> (38.9524, 6.1253) centre (37.5, 6.5003) ccw
  arc A377 (39.4365, 6.5003) -> (38.9524, 6.1253) centre (39.4365, 6.0003) ccw
  line L44 (39.4365, 6.5003) -> (40.5635, 6.5003)
  arc A378 (41.0476, 6.1253) -> (40.5635, 6.5003) centre (40.5635, 6.0003) ccw
  arc A379 (41.0476, 6.1253) -> (42.0833, 5.0594) centre (42.5, 6.5003) ccw
  arc A380 (42.9167, 5.0594) -> (42.0833, 5.0594) centre (42.5, 4.3377) ccw
  arc A381 (42.9167, 5.0594) -> (43.9524, 6.1253) centre (42.5, 6.5003) ccw
  arc A382 (44.4365, 6.5003) -> (43.9524, 6.1253) centre (44.4365, 6.0003) ccw
  line L45 (44.4365, 6.5003) -> (45.5635, 6.5003)
  arc A383 (46.0476, 6.1253) -> (45.5635, 6.5003) centre (45.5635, 6.0003) ccw
  arc A384 (46.0476, 6.1253) -> (47.0833, 5.0594) centre (47.5, 6.5003) ccw
  arc A385 (47.9167, 5.0594) -> (47.0833, 5.0594) centre (47.5, 4.3377) ccw
  arc A386 (47.9167, 5.0594) -> (48.9524, 6.1253) centre (47.5, 6.5003) ccw
  arc A387 (49.2562, 6.4667) -> (48.9524, 6.1253) centre (49.4365, 6.0003) ccw
  arc A388 (50.5422, 6.3993) -> (49.2562, 6.4667) centre (47.5, -39.3462) ccw
  arc A389 (50.8087, 6.028) -> (50.5422, 6.3993) centre (50.3141, 5.9543) ccw
  arc A390 (50.8087, 6.028) -> (51.7273, 4.8596) centre (52.2923, 6.2492) ccw
  arc A391 (52.556, 4.7725) -> (51.7273, 4.8596) centre (52.0662, 4.0984) ccw
  arc A392 (52.556, 4.7725) -> (53.6975, 5.7244) centre (52.2923, 6.2492) ccw
  arc A393 (54.0353, 6.0321) -> (53.6975, 5.7244) centre (54.1659, 5.5495) ccw
  arc A394 (55.3072, 5.8307) -> (54.0353, 6.0321) centre (47.5, -39.3462) ccw
  arc A395 (55.5334, 5.4336) -> (55.3072, 5.8307) centre (55.0339, 5.412) ccw
  arc A396 (55.5334, 5.4336) -> (56.3249, 4.1756) centre (57.032, 5.4985) ccw
  arc A397 (57.14, 4.0024) -> (56.3249, 4.1756) centre (56.5824, 3.3831) ccw
  arc A398 (57.14, 4.0024) -> (58.3747, 4.8297) centre (57.032, 5.4985) ccw
  arc A399 (58.7428, 5.1004) -> (58.3747, 4.8297) centre (58.8222, 4.6068) ccw
  arc A400 (59.9867, 4.7671) -> (58.7428, 5.1004) centre (47.5, -39.3462) ccw
  arc A401 (60.1702, 4.3486) -> (59.9867, 4.7671) centre (59.6711, 4.3793) ccw
  arc A402 (60.1702, 4.3486) -> (60.8258, 3.0148) centre (61.6673, 4.2564) ccw
  arc A403 (61.6183, 2.7572) -> (60.8258, 3.0148) centre (60.999, 2.1996) ccw
  arc A404 (61.6183, 2.7572) -> (62.9327, 3.451) centre (61.6673, 4.2564) ccw
  arc A405 (63.3272, 3.6817) -> (62.9327, 3.451) centre (63.3545, 3.1825) ccw
  arc A406 (64.5294, 3.2202) -> (63.3272, 3.6817) centre (47.5, -39.3462) ccw
  arc A407 (64.6681, 2.7848) -> (64.5294, 3.2202) centre (64.175, 2.8676) ccw
  arc A408 (64.6681, 2.7848) -> (65.1807, 1.3898) centre (66.1474, 2.5367) ccw
  arc A409 (65.942, 1.0508) -> (65.1807, 1.3898) centre (65.2678, 0.561) ccw
  arc A410 (65.942, 1.0508) -> (67.3217, 1.6034) centre (66.1474, 2.5367) ccw
  arc A411 (67.7381, 1.7916) -> (67.3217, 1.6034) centre (67.7131, 1.2923) ccw
  arc A412 (68.8855, 1.207) -> (67.7381, 1.7916) centre (47.5, -39.3462) ccw
  arc A413 (68.978, 0.7595) -> (68.8855, 1.207) centre (68.4962, 0.8933) ccw
  arc A414 (68.978, 0.7595) -> (69.3419, -0.6815) centre (70.4232, 0.3581) ccw
  arc A415 (70.0636, -1.0982) -> (69.3419, -0.6815) centre (69.3419, -1.5149) ccw
  arc A416 (70.0636, -1.0982) -> (71.4935, -0.6929) centre (70.4232, 0.3581) ccw
  arc A417 (71.9273, -0.5492) -> (71.4935, -0.6929) centre (71.8503, -1.0432) ccw
  arc A418 (73.0073, -1.2505) -> (71.9273, -0.5492) centre (47.5, -39.3462) ccw
  arc A419 (73.0525, -1.7053) -> (73.0073, -1.2505) centre (72.5873, -1.5218) ccw
  arc A420 (73.0525, -1.7053) -> (73.2638, -3.1764) centre (74.4479, -2.2556) ccw
  arc A421 (73.938, -3.6663) -> (73.2638, -3.1764) centre (73.1767, -4.0052) ccw
  arc A422 (73.938, -3.6663) -> (75.4025, -3.4126) centre (74.4479, -2.2556) ccw
  arc A423 (75.8489, -3.315) -> (75.4025, -3.4126) centre (75.7206, -3.7983) ccw
  arc A424 (76.8497, -4.1255) -> (75.8489, -3.315) centre (47.5, -39.3462) ccw
  arc A425 (76.847, -4.5824) -> (76.8497, -4.1255) centre (76.4036, -4.3514) ccw
  arc A426 (76.847, -4.5824) -> (76.9034, -6.0676) centre (78.1773, -5.2756) ccw
  arc A427 (77.5227, -6.6252) -> (76.9034, -6.0676) centre (76.7302, -6.8828) ccw
  arc A428 (77.5227, -6.6252) -> (79.0057, -6.5261) centre (78.1773, -5.2756) ccw
  arc A429 (79.4599, -6.4757) -> (79.0057, -6.5261) centre (79.2818, -6.9429) ccw
  arc A430 (80.3705, -7.3863) -> (79.4599, -6.4757) centre (47.5, -39.3462) ccw
  arc A431 (80.3201, -7.8405) -> (80.3705, -7.3863) centre (79.9032, -7.5643) ccw
  arc A432 (80.3201, -7.8405) -> (80.2209, -9.3234) centre (81.5706, -8.6689) ccw
  arc A433 (80.7785, -9.9427) -> (80.2209, -9.3234) centre (79.9634, -10.116) ccw
  arc A434 (80.7785, -9.9427) -> (82.2637, -9.9991) centre (81.5706, -8.6689) ccw
  arc A435 (82.7207, -9.9965) -> (82.2637, -9.9991) centre (82.4948, -10.4425) ccw
  arc A436 (83.5311, -10.9973) -> (82.7207, -9.9965) centre (47.5, -39.3462) ccw
  arc A437 (83.4335, -11.4437) -> (83.5311, -10.9973) centre (83.0478, -11.1255) ccw
  arc A438 (83.4335, -11.4437) -> (83.1799, -12.9082) centre (84.5906, -12.3983) ccw
  arc A439 (83.6697, -13.5823) -> (83.1799, -12.9082) centre (82.841, -13.6695) ccw
  arc A440 (83.6697, -13.5823) -> (85.1409, -13.7937) centre (84.5906, -12.3983) ccw
  arc A441 (85.5956, -13.8388) -> (85.1409, -13.7937) centre (85.3243, -14.2588) ccw
  arc A442 (86.297, -14.9189) -> (85.5956, -13.8388) centre (47.5, -39.3462) ccw
  arc A443 (86.1533, -15.3526) -> (86.297, -14.9189) centre (85.803, -14.9959) ccw
  arc A444 (86.1533, -15.3526) -> (85.748, -16.7826) centre (87.2042, -16.4229) ccw
  arc A445 (86.1646, -17.5042) -> (85.748, -16.7826) centre (85.3313, -17.5042) ccw
  arc A446 (86.1646, -17.5042) -> (87.6056, -17.8682) centre (87.2042, -16.4229) ccw
  arc A447 (88.0532, -17.9606) -> (87.6056, -17.8682) centre (87.7395, -18.35) ccw
  arc A448 (88.6378, -19.1081) -> (88.0532, -17.9606) centre (47.5, -39.3462) ccw
  arc A449 (88.4495, -19.5244) -> (88.6378, -19.1081) centre (88.1384, -19.133) ccw
  arc A450 (88.4495, -19.5244) -> (87.897, -20.9042) centre (89.3828, -20.6987) ccw
  arc A451 (88.2359, -21.6655) -> (87.897, -20.9042) centre (87.4072, -21.5783) ccw
  arc A452 (88.2359, -21.6655) -> (89.631, -22.178) centre (89.3828, -20.6987) ccw
  arc A453 (90.0664, -22.3167) -> (89.631, -22.178) centre (89.7137, -22.6712) ccw
  arc A454 (90.5279, -23.519) -> (90.0664, -22.3167) centre (47.5, -39.3462) ccw
  arc A455 (90.2971, -23.9134) -> (90.5279, -23.519) centre (90.0287, -23.4916) ccw
  arc A456 (90.2971, -23.9134) -> (89.6034, -25.2278) centre (91.1026, -25.1788) ccw
  arc A457 (89.8609, -26.0204) -> (89.6034, -25.2278) centre (89.0458, -25.8471) ccw
  arc A458 (89.8609, -26.0204) -> (91.1948, -26.676) centre (91.1026, -25.1788) ccw
  arc A459 (91.6133, -26.8594) -> (91.1948, -26.676) centre (91.2255, -27.175) ccw
  arc A460 (91.9466, -28.1033) -> (91.6133, -26.8594) centre (47.5, -39.3462) ccw
  arc A461 (91.6759, -28.4715) -> (91.9466, -28.1033) centre (91.4529, -28.0239) ccw
  arc A462 (91.6759, -28.4715) -> (90.8485, -29.7062) centre (92.3446, -29.8141) ccw
  arc A463 (91.0218, -30.5213) -> (90.8485, -29.7062) centre (90.2292, -30.2638) ccw
  arc A464 (91.0218, -30.5213) -> (92.2798, -31.3127) centre (92.3446, -29.8141) ccw
  arc A465 (92.6768, -31.5389) -> (92.2798, -31.3127) centre (92.2582, -31.8123) ccw
  arc A466 (92.8783, -32.8109) -> (92.6768, -31.5389) centre (47.5, -39.3462) ccw
  arc A467 (92.5706, -33.1487) -> (92.8783, -32.8109) centre (92.3957, -32.6803) ccw
  arc A468 (92.5706, -33.1487) -> (91.6187, -34.2901) centre (93.0953, -34.5539) ccw
  arc A469 (91.7058, -35.1189) -> (91.6187, -34.2901) centre (90.9445, -34.78) ccw
  arc A470 (91.7058, -35.1189) -> (92.8742, -36.0375) centre (93.0953, -34.5539) ccw
  arc A471 (93.2454, -36.304) -> (92.8742, -36.0375) centre (92.8005, -36.532) ccw
  arc A472 (93.3128, -37.59) -> (93.2454, -36.304) centre (47.5, -39.3462) ccw
  arc A473 (92.9715, -37.8938) -> (93.3128, -37.59) centre (92.8465, -37.4097) ccw
  arc A474 (92.9715, -37.8938) -> (91.9055, -38.9295) centre (93.3465, -39.3462) ccw
  arc A475 (91.9055, -39.7628) -> (91.9055, -38.9295) centre (91.1838, -39.3462) ccw
  arc A476 (91.9055, -39.7628) -> (92.9715, -40.7985) centre (93.3465, -39.3462) ccw
  arc A477 (93.3128, -41.1023) -> (92.9715, -40.7985) centre (92.8465, -41.2827) ccw
  arc A478 (93.2454, -42.3884) -> (93.3128, -41.1023) centre (47.5, -39.3462) ccw
  arc A479 (92.8742, -42.6548) -> (93.2454, -42.3884) centre (92.8005, -42.1603) ccw
  arc A480 (92.8742, -42.6548) -> (91.7058, -43.5734) centre (93.0953, -44.1384) ccw
  arc A481 (91.6187, -44.4022) -> (91.7058, -43.5734) centre (90.9445, -43.9124) ccw
  arc A482 (91.6187, -44.4022) -> (92.5706, -45.5436) centre (93.0953, -44.1384) ccw
  arc A483 (92.8783, -45.8815) -> (92.5706, -45.5436) centre (92.3957, -46.012) ccw
  arc A484 (92.6768, -47.1534) -> (92.8783, -45.8815) centre (47.5, -39.3462) ccw
  arc A485 (92.2798, -47.3796) -> (92.6768, -47.1534) centre (92.2582, -46.88) ccw
  arc A486 (92.2798, -47.3796) -> (91.0218, -48.171) centre (92.3446, -48.8782) ccw
  arc A487 (90.8485, -48.9861) -> (91.0218, -48.171) centre (90.2292, -48.4285) ccw
  arc A488 (90.8485, -48.9861) -> (91.6759, -50.2208) centre (92.3446, -48.8782) ccw
  arc A489 (91.9466, -50.589) -> (91.6759, -50.2208) centre (91.4529, -50.6684) ccw
  arc A490 (91.6133, -51.8329) -> (91.9466, -50.589) centre (47.5, -39.3462) ccw
  arc A491 (91.1948, -52.0163) -> (91.6133, -51.8329) centre (91.2255, -51.5173) ccw
  arc A492 (91.1948, -52.0163) -> (89.8609, -52.6719) centre (91.1026, -53.5135) ccw
  arc A493 (89.6034, -53.4645) -> (89.8609, -52.6719) centre (89.0458, -52.8452) ccw
  arc A494 (89.6034, -53.4645) -> (90.2971, -54.7789) centre (91.1026, -53.5135) ccw
  arc A495 (90.5279, -55.1733) -> (90.2971, -54.7789) centre (90.0287, -55.2007) ccw
  arc A496 (90.0664, -56.3756) -> (90.5279, -55.1733) centre (47.5, -39.3462) ccw
  arc A497 (89.631, -56.5143) -> (90.0664, -56.3756) centre (89.7137, -56.0212) ccw
  arc A498 (89.631, -56.5143) -> (88.2359, -57.0269) centre (89.3828, -57.9936) ccw
  arc A499 (87.897, -57.7882) -> (88.2359, -57.0269) centre (87.4072, -57.114) ccw
  arc A500 (87.897, -57.7882) -> (88.4495, -59.1679) centre (89.3828, -57.9936) ccw
  arc A501 (88.6378, -59.5843) -> (88.4495, -59.1679) centre (88.1384, -59.5593) ccw
  arc A502 (88.0532, -60.7317) -> (88.6378, -59.5843) centre (47.5, -39.3462) ccw
  arc A503 (87.6056, -60.8241) -> (88.0532, -60.7317) centre (87.7395, -60.3424) ccw
  arc A504 (87.6056, -60.8241) -> (86.1646, -61.1881) centre (87.2042, -62.2694) ccw
  arc A505 (85.748, -61.9098) -> (86.1646, -61.1881) centre (85.3313, -61.1881) ccw
  arc A506 (85.748, -61.9098) -> (86.1533, -63.3397) centre (87.2042, -62.2694) ccw
  arc A507 (86.297, -63.7735) -> (86.1533, -63.3397) centre (85.803, -63.6965) ccw
  arc A508 (85.5956, -64.8535) -> (86.297, -63.7735) centre (47.5, -39.3462) ccw
  arc A509 (85.1409, -64.8986) -> (85.5956, -64.8535) centre (85.3243, -64.4335) ccw
  arc A510 (85.1409, -64.8986) -> (83.6697, -65.11) centre (84.5906, -66.294) ccw
  arc A511 (83.1799, -65.7842) -> (83.6697, -65.11) centre (82.841, -65.0229) ccw
  arc A512 (83.1799, -65.7842) -> (83.4335, -67.2486) centre (84.5906, -66.294) ccw
  arc A513 (83.5311, -67.695) -> (83.4335, -67.2486) centre (83.0478, -67.5668) ccw
  arc A514 (82.7207, -68.6958) -> (83.5311, -67.695) centre (47.5, -39.3462) ccw
  arc A515 (82.2637, -68.6932) -> (82.7207, -68.6958) centre (82.4948, -68.2498) ccw
  arc A516 (82.2637, -68.6932) -> (80.7785, -68.7496) centre (81.5706, -70.0234) ccw
  arc A517 (80.2209, -69.3689) -> (80.7785, -68.7496) centre (79.9634, -68.5763) ccw
  arc A518 (80.2209, -69.3689) -> (80.3201, -70.8518) centre (81.5706, -70.0234) ccw
  arc A519 (80.3705, -71.306) -> (80.3201, -70.8518) centre (79.9032, -71.128) ccw
  arc A520 (79.4599, -72.2166) -> (80.3705, -71.306) centre (47.5, -39.3462) ccw
  arc A521 (79.0057, -72.1662) -> (79.4599, -72.2166) centre (79.2818, -71.7494) ccw
  arc A522 (79.0057, -72.1662) -> (77.5227, -72.0671) centre (78.1773, -73.4167) ccw
  arc A523 (76.9034, -72.6247) -> (77.5227, -72.0671) centre (76.7302, -71.8096) ccw
  arc A524 (76.9034, -72.6247) -> (76.847, -74.1099) centre (78.1773, -73.4167) ccw
  arc A525 (76.8497, -74.5668) -> (76.847, -74.1099) centre (76.4036, -74.3409) ccw
  arc A526 (75.8489, -75.3773) -> (76.8497, -74.5668) centre (47.5, -39.3462) ccw
  arc A527 (75.4025, -75.2797) -> (75.8489, -75.3773) centre (75.7206, -74.894) ccw
  arc A528 (75.4025, -75.2797) -> (73.938, -75.0261) centre (74.4479, -76.4367) ccw
  arc A529 (73.2638, -75.5159) -> (73.938, -75.0261) centre (73.1767, -74.6871) ccw
  arc A530 (73.2638, -75.5159) -> (73.0525, -76.987) centre (74.4479, -76.4367) ccw
  arc A531 (73.0073, -77.4418) -> (73.0525, -76.987) centre (72.5873, -77.1705) ccw
  arc A532 (71.9273, -78.1432) -> (73.0073, -77.4418) centre (47.5, -39.3462) ccw
  arc A533 (71.4935, -77.9994) -> (71.9273, -78.1432) centre (71.8503, -77.6491) ccw
  arc A534 (71.4935, -77.9994) -> (70.0636, -77.5941) centre (70.4232, -79.0504) ccw
  arc A535 (69.3419, -78.0108) -> (70.0636, -77.5941) centre (69.3419, -77.1775) ccw
  arc A536 (69.3419, -78.0108) -> (68.978, -79.4518) centre (70.4232, -79.0504) ccw
  arc A537 (68.8855, -79.8993) -> (68.978, -79.4518) centre (68.4962, -79.5856) ccw
  arc A538 (67.7381, -80.484) -> (68.8855, -79.8993) centre (47.5, -39.3462) ccw
  arc A539 (67.3217, -80.2957) -> (67.7381, -80.484) centre (67.7131, -79.9846) ccw
  arc A540 (67.3217, -80.2957) -> (65.942, -79.7431) centre (66.1474, -81.229) ccw
  arc A541 (65.1807, -80.0821) -> (65.942, -79.7431) centre (65.2678, -79.2533) ccw
  arc A542 (65.1807, -80.0821) -> (64.6681, -81.4772) centre (66.1474, -81.229) ccw
  arc A543 (64.5294, -81.9126) -> (64.6681, -81.4772) centre (64.175, -81.5599) ccw
  arc A544 (63.3272, -82.3741) -> (64.5294, -81.9126) centre (47.5, -39.3462) ccw
  arc A545 (62.9327, -82.1433) -> (63.3272, -82.3741) centre (63.3545, -81.8748) ccw
  arc A546 (62.9327, -82.1433) -> (61.6183, -81.4496) centre (61.6673, -82.9488) ccw
  arc A547 (60.8258, -81.7071) -> (61.6183, -81.4496) centre (60.999, -80.8919) ccw